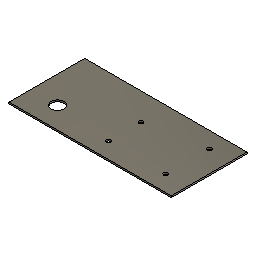
NixieRückwand (Autodesk Fusion 360 design; units mm, degrees)
Autodesk Fusion 360 part; units mm, degrees
sketch "Skizze1" plane through (0, 0, 0) normal (0, 1, 0) x (1, 0, 0)
  line L0 (0, 0) -> (150, 0)
  line L1 (150, 0) -> (150, 70)
  line L2 (150, 70) -> (0, 70)
  line L3 (0, 70) -> (0, 0)
  dimension "d1" = 150
  dimension "d2" = 70
  constraint horizontal L0
  constraint vertical L1
  constraint horizontal L2
  constraint vertical L3
  constraint coincident L0.start L3.end
  measures "d1" distance of L0.start L0.end
  measures "d2" distance of L0.start L2.end
extrude "Extrusion1" add sketch "Skizze1" along normal blind 1.5
sketch "Skizze2" plane through (0, 1.5, 0) normal (0, 1, 0) x (-1, 0, 0)
  line L0 (0, -70) -> (0, 0)
  line L1 (0, 0) -> (-150, 0)
  line L2 (-150, 0) -> (-150, -70)
  line L3 (-150, -70) -> (0, -70)
  line L4 (-77, -55) -> (-130, -55) construction
  line L5 (-130, -55) -> (-130, -15) construction
  line L6 (-130, -15) -> (-77, -15) construction
  line L7 (-77, -15) -> (-77, -55) construction
  line L8 (-81.1558, -15) -> (-81.1558, -45) construction
  circle A0 centre (-130, -55) radius 2
  circle A1 centre (-77, -45) radius 2
  circle A2 centre (-77, -15) radius 2
  circle A3 centre (-130, -15) radius 2
  circle A4 centre (-25, -20) radius 6
  dimension "d5" = 53
  dimension "d6" = 40
  dimension "d7" = 20
  dimension "d8" = 15
  dimension "d10" = 4
  dimension "d11" = 4
  dimension "d12" = 4
  dimension "d13" = 4
  dimension "d14" = 12
  dimension "d17" = 30
  constraint horizontal L4
  constraint vertical L5
  constraint horizontal L6
  constraint vertical L7
  constraint coincident L6 L8.start
  constraint perpendicular L6 L8
  constraint coincident L4.end L5.start
  constraint coincident L7 A1.centre
  constraint coincident L6.end L7.start
  constraint coincident L5.end L6.start
  measures "d5" distance of L4.start L4.end
  measures "d6" distance of L4.start L6.end
  measures "d7" distance of L2 L5
  measures "d8" distance of L1 L6
  measures "d10" diameter of A0
  measures "d11" diameter of A1
  measures "d12" diameter of A2
  measures "d13" diameter of A3
  measures "d14" diameter of A4
  measures "d17" distance of A1.centre L6.end
extrude "Extrusion2" cut sketch "Skizze2" against normal blind 5 contours A0 | A1 | A2 | A3 | A4
